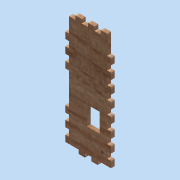
# Autodesk Inventor part: Right_wall
Saved by Autodesk Inventor 2015 (Build 190159000, 159)
## iProperties
Created: 2015-01-31
Part Number: Right_wall
Material: Wood (Birch)
Document SubType Name: Modeling
Designer: Openlab
Density: 0.55 g/cm^3
Appearance: Birch - Natural Polished
Author: Openlab
Autodesk Inventor part; units mm, degrees
ref_plane "YZ Plane" through (0, 0, 0) normal (1, 0, 0) x (0, 1, 0)
ref_plane "XZ Plane" through (0, 0, 0) normal (0, 1, 0) x (-1, 0, 0)
ref_plane "XY Plane" through (0, 0, 0) normal (0, 0, 1) x (1, 0, 0)
sketch "Sketch1" plane through (0, 0, 0) normal (0, 1, 0) x (-1, 0, 0)
  line L0 (-30, -15) -> (-33, -15)
  line L1 (-33, -15) -> (-33, -20)
  line L2 (-33, -20) -> (-30, -20)
  line L3 (-30, 0) -> (-30, -15)
  line L4 (-30, -25) -> (-33, -25)
  line L5 (-33, -25) -> (-33, -30)
  line L6 (-33, -30) -> (-30, -30)
  line L7 (-30, -35) -> (-33, -35)
  line L8 (-33, -35) -> (-33, -40)
  line L9 (-33, -40) -> (-30, -40)
  line L10 (-30, -45) -> (-33, -45)
  line L11 (-33, -45) -> (-33, -50)
  line L12 (-33, -50) -> (-30, -50)
  line L13 (-30, -55) -> (-33, -55)
  line L14 (-33, -55) -> (-33, -60)
  line L15 (-33, -60) -> (-30, -60)
  line L16 (-30, -65) -> (-33, -65)
  line L17 (-33, -65) -> (-33, -70)
  line L18 (-33, -70) -> (-30, -70)
  line L19 (-30, -75) -> (-33, -75)
  line L20 (-33, -75) -> (-33, -80)
  line L21 (-33, -80) -> (-30, -80)
  line L22 (-30, -20) -> (-30, -25)
  line L23 (-30, -30) -> (-30, -35)
  line L24 (-30, -40) -> (-30, -45)
  line L25 (-30, -50) -> (-30, -55)
  line L26 (-30, -60) -> (-30, -65)
  line L27 (-30, -70) -> (-30, -75)
  line L28 (0, -15) -> (3, -15)
  line L29 (3, -15) -> (3, -20)
  line L30 (3, -20) -> (0, -20)
  line L31 (0, -15) -> (0, -3)
  line L32 (0, -25) -> (3, -25)
  line L33 (3, -25) -> (3, -30)
  line L34 (3, -30) -> (0, -30)
  line L35 (0, -35) -> (3, -35)
  line L36 (3, -35) -> (3, -40)
  line L37 (3, -40) -> (0, -40)
  line L38 (0, -65) -> (3, -65)
  line L39 (3, -65) -> (3, -70)
  line L40 (3, -70) -> (0, -70)
  line L41 (0, -75) -> (3, -75)
  line L42 (3, -75) -> (3, -80)
  line L43 (3, -80) -> (0, -80)
  line L44 (0, -25) -> (0, -20)
  line L45 (0, -35) -> (0, -30)
  line L46 (0, -65) -> (0, -40)
  line L47 (0, -75) -> (0, -70)
  line L48 (-25, 0) -> (-25, -3)
  line L49 (-25, -3) -> (-20, -3)
  line L50 (-20, -3) -> (-20, 0)
  line L51 (-25, 0) -> (-30, 0)
  line L52 (-15, 0) -> (-15, -3)
  line L53 (-15, -3) -> (-10, -3)
  line L54 (-10, -3) -> (-10, 0)
  line L55 (-5, 0) -> (-5, -3)
  line L56 (-5, -3) -> (0, -3)
  line L57 (-5, 0) -> (-10, 0)
  line L58 (-15, 0) -> (-20, 0)
  line L59 (0, -85) -> (3, -85)
  line L60 (3, -85) -> (3, -90)
  line L61 (3, -90) -> (0, -90)
  line L62 (-30, -85) -> (-33, -85)
  line L63 (-33, -85) -> (-33, -90)
  line L64 (-33, -90) -> (-30, -90)
  line L65 (0, -85) -> (0, -80)
  line L66 (-30, -80) -> (-30, -85)
  line L67 (-7.5, -90) -> (-7.5, -93)
  line L68 (-7.5, -93) -> (-12.5, -93)
  line L69 (-12.5, -93) -> (-12.5, -90)
  line L70 (-22.5, -90) -> (-22.5, -93)
  line L71 (-22.5, -93) -> (-17.5, -93)
  line L72 (-17.5, -93) -> (-17.5, -90)
  line L73 (0, -90) -> (-7.5, -90)
  line L74 (-12.5, -90) -> (-17.5, -90)
  line L75 (-22.5, -90) -> (-30, -90)
  line L76 (-24, -63.5) -> (-10, -63.5) construction
  line L77 (-24.0357, -71) -> (-24.0357, -56)
  line L78 (-24.0357, -56) -> (-14.0357, -56)
  line L79 (-14.0357, -56) -> (-14.0357, -71)
  line L80 (-14.0357, -71) -> (-24.0357, -71)
  point P0 (0, 0)
  dimension "d11" = 10
  dimension "d14" = 10
  dimension "d22" = 10
  dimension "d25" = 10
  dimension "d2" = 15
  dimension "d3" = 5
  dimension "d4" = 3
  dimension "d16" = 15
  dimension "d17" = 5
  dimension "d19" = 3
  dimension "d27" = 30
  dimension "d28" = 3
  dimension "d29" = 5
  dimension "d30" = 3
  dimension "d31" = 7.5
  dimension "d32" = 29.5
  dimension "d33" = 5.9643
  dimension "d34" = 10
  dimension "d35" = 15
  dimension "d38" = 25
  constraints: 162 end point, 51 perpendicular, 29 equal length, 28 collinear, 6 horizontal, 6 point on line, 2 vertical, 1 horizontal alignment, 1 parallel, 1 vertical alignment, 1 other
  measures "d2" distance of L3.start L0.start
  measures "d3" distance of L0.end L1.end
  measures "d4" distance of L0.start L0.end
  measures "d16" distance of L28.start point (0, 0)
  measures "d17" distance of L28.end L29.end
  measures "d19" distance of L28.start L28.end
  measures "d27" distance of point (0, 0) L3.start
  measures "d28" distance of L55.start L55.end
  measures "d29" distance of L55.end L31.end
  measures "d30" distance of L70.start L70.end
  measures "d31" distance between parallel lines of L66 L70
  measures "d32" distance between parallel lines of L76 L71
  measures "d33" distance between parallel lines of L26 L77
  measures "d34" distance of L77.end L78.end
  measures "d35" distance of L78.end L79.end
  measures "d38" distance of L38.start L37.end
extrude "Extrusion2" add sketch "Sketch1" along normal blind 3
equation "\"d4\" = x"
equation "\"d19\" = x"
equation "\"d28\" = x"
equation "\"d30\" = x"
equation "\"x\" = 3"
body "Solid2"
